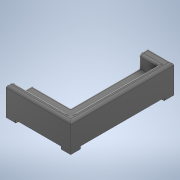
# Autodesk Inventor part: couch
Saved by Autodesk Inventor 2022 (Build 260153000, 153)
## iProperties
Created: 2022-05-13
Part Number: couch
Material: Generic
Document SubType Name: Modeling
Designer: mihir
Density: 1 g/cm^3
Appearance: Default
Author: mihir
Autodesk Inventor part; units mm, degrees
ref_plane "YZ Plane" through (0, 0, 0) normal (1, 0, 0) x (0, 1, 0)
ref_plane "XZ Plane" through (0, 0, 0) normal (0, 1, 0) x (-1, 0, 0)
ref_plane "XY Plane" through (0, 0, 0) normal (0, 0, 1) x (1, 0, 0)
sketch "Sketch1" plane through (0, 0, 0) normal (0, 1, 0) x (-1, 0, 0)
  line L0 (50, 0) -> (0, 0)
  line L1 (0, 0) -> (0, -20)
  line L2 (0, -20) -> (50, -20)
  line L3 (50, -20) -> (50, 0)
  line L4 (0, 0) -> (20, 0)
  line L5 (20, 0) -> (20, -80)
  line L6 (20, -80) -> (0, -80)
  line L7 (0, -80) -> (0, 0)
  point P0 (0, 0)
  point P1 (20, -20)
  dimension "d0" = 50
  dimension "d1" = 20
  dimension "d2" = 80
  dimension "d3" = 20
  dimension "d4" = 0
  dimension "d5" = 0
  constraints: 16 end point, 4 parallel, 2 horizontal, 2 perpendicular
  measures "d0" distance of L2.end L1.end
  measures "d1" distance of L5.end L6.end
  measures "d2" distance of L4.end L5.end
  measures "d3" distance of L2.end L0.start
  measures "d4" distance from line of point (0, 0) L1
  measures "d5" distance from line of point (0, 0) L0
extrude "Extrusion1" add sketch "Sketch1" along normal blind 10
sketch "Sketch3" plane through (0, 10, 0) normal (0, 1, 0) x (1, 0, 0)
  line L0 (0, 80) -> (-20, 80) projected
  line L1 (-20, 80) -> (0, 80)
  line L2 (0, 80) -> (0, 72.5)
  line L3 (0, 72.5) -> (-20, 72.5)
  line L4 (-20, 72.5) -> (-20, 80)
  line L5 (0, 0) -> (0, 80) projected
  line L6 (0, 80) -> (-5, 80)
  line L7 (-5, 80) -> (-5, 0)
  line L8 (-5, 0) -> (0, 0)
  line L9 (0, 0) -> (0, 80)
  line L10 (-50, 20) -> (-50, 0) projected
  line L11 (0, 0) -> (-50, 0)
  line L12 (0, 10) -> (0, 0)
  line L13 (-50, 0) -> (0, 0) projected
  line L14 (0, 0) -> (-50, 0)
  line L15 (-50, 0) -> (-50, 5)
  line L16 (-50, 5) -> (0, 5)
  line L17 (0, 5) -> (0, 0)
  point P0 (-50, 10)
  point P1 (-5, 72.5)
  point P2 (-5, 5)
  point P3 (-5, 0)
  dimension "d8" = 20
  dimension "d9" = 7.5
  dimension "d10" = 5
  dimension "d11" = 80
  dimension "d14" = 50
  dimension "d15" = 5
  constraints: 28 end point, 6 parallel, 4 horizontal, 3 perpendicular, 1 midpoint
  measures "d8" distance of L2.end L3.end
  measures "d9" distance of L1.end L2.end
  measures "d10" distance of L8.end L7.end
  measures "d11" distance of L7.end L6.end
  measures "d14" distance of L15.end L16.end
  measures "d15" distance of L14.end L15.end
extrude "Extrusion2" add sketch "Sketch3" along normal blind 10 contours L2 L3 L7 L0 | L7 L3 L4 L0 | L5 L16 L7 L3 | L16 L5 L8 L7
extrude "Extrusion3" add sketch "Sketch3" along normal blind 10 contours L7 L11 L10 L16
fillet "Fillet1" radius 2 16 edges at (-5, 20, -38.75) (-5, 10, -38.75) (-27.5, 20, -5) (-27.5, 10, -5) (-5, 15, -5) (-20, 10, -46.25) (-35, 10, -20) (-12.5, 20, -72.5) (-10, 20, -80) (-20, 20, -76.25) (-20, 15, -72.5) (-50, 10, -12.5) (-50, 15, -5) (-50, 20, -2.5) (0, 20, -40) (-25, 20, 0)
sketch "Sketch4" plane through (0, 0, 0) normal (0, -1, 0) x (1, 0, 0)
  line L0 (0, 0) -> (-7.5, 0)
  line L1 (-7.5, 0) -> (-7.5, -7.5)
  line L2 (-7.5, -7.5) -> (0, -7.5)
  line L3 (0, -7.5) -> (0, 0)
  line L4 (-20, -20) -> (-50, -20) projected
  line L5 (-50, -20) -> (-42.5, -20)
  line L6 (-42.5, -20) -> (-42.5, -12.5)
  line L7 (-42.5, -12.5) -> (-50, -12.5)
  line L8 (-50, -12.5) -> (-50, -20)
  line L9 (-50, 0) -> (0, 0) projected
  line L10 (-50, 0) -> (-42.5, 0)
  line L11 (-42.5, 0) -> (-42.5, -7.5)
  line L12 (-42.5, -7.5) -> (-50, -7.5)
  line L13 (-50, -7.5) -> (-50, 0)
  line L14 (-18, -18) -> (-20, -20) projected
  line L15 (-20, -20) -> (-12.3, -20)
  line L16 (-12.3, -20) -> (-12.3, -12.5)
  line L17 (-12.3, -12.5) -> (-20, -12.5)
  line L18 (-20, -12.5) -> (-20, -20)
  line L19 (0, -80) -> (-20, -80) projected
  line L20 (-20, -80) -> (-12.5, -80)
  line L21 (-12.5, -80) -> (-12.5, -72.5)
  line L22 (-12.5, -72.5) -> (-20, -72.5)
  line L23 (-20, -72.5) -> (-20, -80)
  line L24 (0, 0) -> (0, -80) projected
  line L25 (0, -80) -> (-7.5, -80)
  line L26 (-7.5, -80) -> (-7.5, -72.5)
  line L27 (-7.5, -72.5) -> (0, -72.5)
  line L28 (0, -72.5) -> (0, -80)
  point P0 (0, -72.5)
  dimension "d19" = 7.5
  dimension "d20" = 7.5
  dimension "d21" = 7.5
  dimension "d22" = 7.5
  dimension "d23" = 7.5
  dimension "d24" = 7.5
  dimension "d25" = 7.7
  dimension "d26" = 7.5
  dimension "d27" = 7.5
  dimension "d28" = 7.5
  dimension "d29" = 7.5
  dimension "d30" = 7.5
  constraints: 48 end point, 12 parallel, 6 horizontal, 6 perpendicular
  measures "d19" distance of L2.end L1.end
  measures "d20" distance of L1.end L0.end
  measures "d21" distance of L7.end L6.end
  measures "d22" distance of L6.end L5.end
  measures "d23" distance of L11.end L12.end
  measures "d24" distance of L10.end L11.end
  measures "d25" distance of L17.end L16.end
  measures "d26" distance of L16.end L15.end
  measures "d27" distance of L22.end L21.end
  measures "d28" distance of L21.end L20.end
  measures "d29" distance of L26.end L27.end
  measures "d30" distance of L25.end L26.end
extrude "Extrusion4" add sketch "Sketch4" along normal blind 2
body "Solid1"
